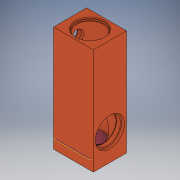
# Autodesk Inventor part: pipeshift
Saved by Autodesk Inventor 2018 (Build 220112000, 112)
## iProperties
Created: 2019-03-06
Part Number: pipeshift
Material: Copper
Document SubType Name: Modeling
Designer: Admin
Density: 8.94 g/cm^3
Appearance: Copper - Satin
Mass: 626.759 g
Surface Area: 238.443 cm^2
Volume: 70.1073 cm^3
Author: Admin
Autodesk Inventor part; units mm, degrees
ref_plane "YZ Plane" through (0, 0, 0) normal (1, 0, 0) x (0, 1, 0)
ref_plane "XZ Plane" through (0, 0, 0) normal (0, 1, 0) x (-1, 0, 0)
ref_plane "XY Plane" through (0, 0, 0) normal (0, 0, 1) x (1, 0, 0)
sketch "Sketch1" plane through (0, 0, 0) normal (0, 1, 0) x (-1, 0, 0)
  line L0 (-19.05, 15.875) -> (19.05, 15.875)
  line L1 (19.05, 15.875) -> (19.05, -15.875)
  line L2 (19.05, -15.875) -> (-19.05, -15.875)
  line L3 (-19.05, -15.875) -> (-19.05, 15.875)
  line L4 (-19.05, 15.875) -> (19.05, -15.875) construction
  line L5 (19.05, 15.875) -> (-19.05, -15.875) construction
  point P0 (0, 0)
  dimension "d0" = 38.1
  dimension "d1" = 31.75
  constraints: 12 end point, 2 midpoint, 2 parallel, 1 horizontal, 1 perpendicular
  measures "d0" distance of L1.end L2.end
  measures "d1" distance between parallel lines of L2 L0
extrude "Extrusion1" add sketch "Sketch1" along normal blind 101.6
ref_plane "Work Plane1" through (0, 10.16, 0) normal (0, -1, 0) x (1, 0, 0)
sketch "Sketch2" plane through (0, 101.6, 0) normal (0, 1, 0) x (1, 0, 0)
  point P0 (0, 0)
  point P1 (0, 0)
  constraints: 1 coincident
hole "Hole1" at (0, 101.6, 0) direction (0, -1, 0) diameter 25.4 depth 91.44 tip angle 118
sketch "Sketch3" plane through (19.05, 0, 15.875) normal (1, 0, 0) x (0, 0, -1)
  line L0 (15.875, 0) -> (15.875, 25.4) construction
  circle A0 centre (15.875, 25.4) radius 13.97
  dimension "d12" = 25.4
  dimension "d13" = 27.94
  constraints: 2 end point, 1 centre point, 1 coincident, 1 vertical
  measures "d12" distance of L0.start L0.end
  measures "d13" diameter of A0
extrude "Extrusion2" cut sketch "Sketch3" against normal blind 2.54
sketch "Sketch5" plane through (19.05, 0, 15.875) normal (1, 0, 0) x (0, 0, -1)
  circle A0 centre (15.875, 25.4) radius 13.97 projected
  circle A1 centre (15.875, 25.4) radius 12.7
  point P0 (15.875, 0)
  dimension "d20" = 25.4
  constraints: 1 centre point, 1 coincident
  measures "d20" diameter of A1
extrude "Extrusion4" cut sketch "Sketch5" against normal blind 6.35 contours A1
sketch "Sketch6" plane through (19.05, 0, 15.875) normal (1, 0, 0) x (0, 0, -1)
  circle A0 centre (15.875, 25.4) radius 13.97 projected
  circle A1 centre (15.875, 25.4) radius 12.319
  point P0 (15.875, 0)
  dimension "d23" = 24.638
  constraints: 1 centre point, 1 coincident
  measures "d23" diameter of A1
extrude "Extrusion5" cut sketch "Sketch6" against normal up to surface contours A1 round surface about axis through (0, -11.4585, 0) along (0, 1, 0) radius 12.7 far side no
sketch "Sketch4" plane through (-19.05, 0, -15.875) normal (-1, 0, 0) x (0, 0, 1)
  line L0 (31.75, 101.6) -> (0, 101.6) projected
  line L1 (15.875, 101.6) -> (15.875, 88.9) construction
  circle A0 centre (15.875, 88.9) radius 5.715
  point P0 (15.875, 0)
  dimension "d16" = 12.7
  dimension "d17" = 11.43
  constraints: 2 end point, 1 centre point, 1 coincident, 1 midpoint, 1 vertical
  measures "d16" distance of L1.start L1.end
  measures "d17" diameter of A0
extrude "Extrusion3" cut sketch "Sketch4" against normal up to surface round surface about axis through (0, -11.4585, 0) along (0, 1, 0) radius 12.7 far side no
sketch "Sketch7" plane through (-19.05, 0, -15.875) normal (-1, 0, 0) x (0, 0, 1)
  circle A0 centre (15.875, 88.9) radius 5.715 projected
  circle A1 centre (15.875, 88.9) radius 6.985
  point P0 (15.875, 0)
  dimension "d26" = 13.97
  constraints: 1 centre point, 1 coincident
  measures "d26" diameter of A1
extrude "Extrusion7" cut sketch "Sketch7" against normal blind 1.27 contours A0 | A1
sketch "Sketch8" plane through (-19.05, 0, -15.875) normal (-1, 0, 0) x (0, 0, 1)
  circle A0 centre (15.875, 88.9) radius 6.985 projected
  circle A1 centre (15.875, 88.9) radius 6.35
  point P0 (15.875, 0)
  dimension "d31" = 12.7
  constraints: 1 centre point, 1 coincident
  measures "d31" diameter of A1
extrude "Extrusion8" cut sketch "Sketch8" against normal blind 5.08 contours A1
sketch "Sketch9" plane through (0, 101.6, 0) normal (0, 1, 0) x (1, 0, 0)
  circle A0 centre (0, 0) radius 13.335
  dimension "d34" = 26.67
  constraints: 1 centre point, 1 coincident
  measures "d34" diameter of A0
extrude "Extrusion9" cut sketch "Sketch9" against normal blind 2.54
sketch "Sketch10" plane through (0, 101.6, 0) normal (0, 1, 0) x (1, 0, 0)
  circle A0 centre (0, 0) radius 13.97
  dimension "d37" = 27.94
  constraints: 1 centre point, 1 coincident
  measures "d37" diameter of A0
extrude "Extrusion10" cut sketch "Sketch10" against normal blind 1.27
body "Solid1"
